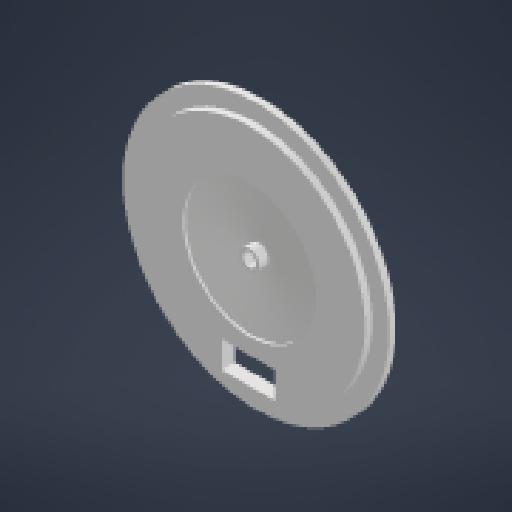
# Autodesk Inventor part: Rotating Plate
Saved by Autodesk Inventor 2023 (Build 270158000, 158)
## iProperties
Created: 2023-04-07
Part Number: Rotating Plate
Material: Generic
Document SubType Name: Modeling
Designer: vatdu
Density: 1 g/cm^3
Appearance: Default
Author: vatdu
Autodesk Inventor part; units mm, degrees
ref_plane "YZ Plane" through (0, 0, 0) normal (1, 0, 0) x (0, 1, 0)
ref_plane "XZ Plane" through (0, 0, 0) normal (0, 1, 0) x (-1, 0, 0)
ref_plane "XY Plane" through (0, 0, 0) normal (0, 0, 1) x (1, 0, 0)
sketch "Sketch1" plane through (0, 0, 0) normal (0, 0, 1) x (1, 0, 0)
  circle A0 centre (0, 0) radius 100
  dimension "d0" = 200
  constraints: 1 centre point, 1 coincident
  measures "d0" diameter of A0
extrude "Extrusion1" add sketch "Sketch1" along normal blind 5
sketch "Sketch2" plane through (0, 0, 5) normal (0, 0, 1) x (1, 0, 0)
  circle A0 centre (0, 0) radius 87
  dimension "d3" = 174
  constraints: 1 centre point, 1 coincident
  measures "d3" diameter of A0
extrude "Extrusion2" add sketch "Sketch2" along normal blind 5
sketch "Sketch3" plane through (0, 0, 10) normal (0, 0, 1) x (1, 0, 0)
  circle A0 centre (0, 0) radius 5
  dimension "d6" = 10
  constraints: 1 centre point, 1 coincident
  measures "d6" diameter of A0
extrude "Extrusion3" cut sketch "Sketch3" against normal blind 10
sketch "Sketch4" plane through (0, 0, 10) normal (0, 0, 1) x (1, 0, 0)
  circle A0 centre (0, 0) radius 7.5
  circle A1 centre (0, 0) radius 5 projected
  circle A2 centre (0, 0) radius 50
  dimension "d9" = 15
  dimension "d10" = 100
  constraints: 2 centre point, 2 coincident
  measures "d9" diameter of A0
  measures "d10" diameter of A2
extrude "Extrusion4" cut sketch "Sketch4" against normal blind 7 contours A2
chamfer "Chamfer1" distance 5 distance2 40 1 edges at (-50, 0, 3) measured on face at (-30.4381, 39.6677, 7.6667)
sketch "Sketch10" plane through (0, 0, 0) normal (0, 0, -1) x (-1, 0, 0)
  circle A0 centre (0, 0) radius 100 projected
  line L0 (0, -100) -> (0, -82.127)
  line L1 (0, -82.127) -> (20.7525, -82.127)
  line L2 (20.7525, -82.127) -> (-19.3985, -82.127)
  line L3 (-19.3985, -82.127) -> (-19.3985, -62.127)
  line L4 (-19.3985, -62.127) -> (20.7525, -62.127)
  line L5 (20.7525, -62.127) -> (20.7525, -82.127)
  dimension "d52" = 17.873
  dimension "d53" = 20.7525
  dimension "d54" = 40.151
  dimension "d55" = 20
  constraints: 12 end point, 3 perpendicular, 1 horizontal, 1 point on line, 1 vertical, 1 vertical alignment, 1 other
  measures "d52" distance of L0.start L0.end
  measures "d53" distance of L0.end L1.end
  measures "d54" distance of L1.end L2.end
  measures "d55" distance of L2.end L3.end
extrude "Extrusion10" cut sketch "Sketch10" against normal blind 10 contours L2 L3 L4 L5 L1
body "Solid1"
